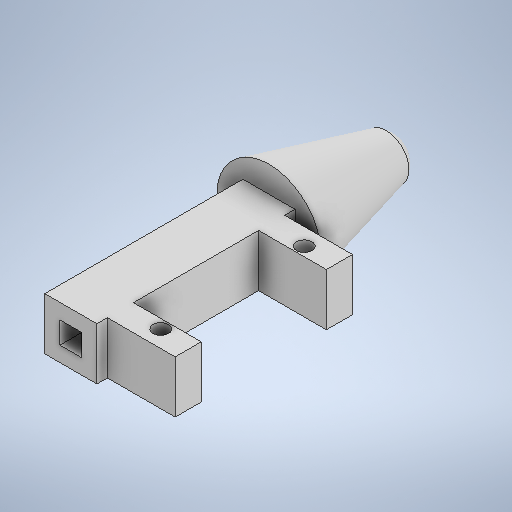
# Autodesk Inventor part: fot
Saved by Autodesk Inventor 2025.1 (Build 291241020, 241B)
## iProperties
Created: 2024-10-04
Part Number: fot
Material: Generic
Document SubType Name: Modeling
Designer: morte
Density: 1 g/cm^3
Appearance: Default
Author: morte
Autodesk Inventor part; units mm, degrees
ref_plane "YZ Plane" through (0, 0, 0) normal (1, 0, 0) x (0, 1, 0)
ref_plane "XZ Plane" through (0, 0, 0) normal (0, 1, 0) x (-1, 0, 0)
sketch "Sketch1" plane through (0, 0, 0) normal (0, 0, 1) x (1, 0, 0)
  line L0 (3.15, -3.15) -> (-3.15, -3.15)
  line L1 (-3.15, -3.15) -> (-3.15, 3.15)
  line L2 (-3.15, 3.15) -> (3.15, 3.15)
  line L3 (3.15, 3.15) -> (3.15, -3.15)
  line L4 (3.15, -3.15) -> (-3.15, 3.15) construction
  line L5 (-3.15, -3.15) -> (3.15, 3.15) construction
  line L6 (5, -5) -> (-5, -5)
  line L7 (-5, -5) -> (-5, 5)
  line L8 (-5, 5) -> (5, 5)
  line L9 (5, 5) -> (5, -5)
  line L10 (5, -5) -> (-5, 5) construction
  line L11 (-5, -5) -> (5, 5) construction
  point P0 (0, 0)
  dimension "d0" = 6.3
  dimension "d1" = 6.3
  dimension "d2" = 10
  dimension "d3" = 10
  constraints: 24 end point, 4 midpoint, 4 parallel, 2 horizontal, 2 perpendicular
  measures "d0" distance of L1.end L2.end
  measures "d1" distance of L0.end L1.end
  measures "d2" distance of L7.end L8.end
  measures "d3" distance of L6.end L7.end
extrude "Extrusion1" add sketch "Sketch1" along normal mid plane 60
sketch "Sketch3" plane through (0, 0, 0) normal (1, 0, 0) x (0, 1, 0)
  line L0 (5, -30) -> (-5, -30) projected
  line L1 (0, -30) -> (0, -50)
  line L2 (0, -30) -> (10, -30)
  arc A0 (0, -55) -> (4.3301, -52.5) centre (0, -50) ccw
  line L3 (0, -55) -> (0, -30)
  line L4 (4.3301, -52.5) -> (10, -30)
  point P0 (0, 0)
  dimension "d19" = 20
  dimension "d20" = 10
  dimension "d21" = 10
  dimension "d22" = 5
  constraints: 8 end point, 2 point on circle, 1 centre point, 1 coincident, 1 midpoint, 1 perpendicular, 1 point on line, 1 vertical
  measures "d19" distance of L1.start L1.end
  measures "d20" distance of L1.start L2.end
  measures "d21" diameter of A0
  measures "d22" distance of L3.start L4.start
revolve "Revolution1" add sketch "Sketch3" angle 360 about axis through (0, 0, -30) along (0, 0, -1)
sketch "Sketch4" plane through (0, 0, 0) normal (0, 1, 0) x (-1, 0, 0)
  point P0 (0, 0)
sketch "Sketch5" plane through (0, 0, 0) normal (0, 1, 0) x (-1, 0, 0)
  line L0 (-5, -30) -> (-5, 30) projected
  line L1 (-5, 0) -> (-5, -23)
  line L2 (-5, 30) -> (-5, -30) projected
  line L3 (-5, 0) -> (-5, 1)
  line L4 (-5, 1) -> (-5, 6)
  line L5 (-5, 6) -> (-18, 6)
  line L6 (-5, -23) -> (-5, -28)
  line L7 (-5, -28) -> (-18, -28)
  line L8 (-18, -28) -> (-18, -23)
  line L9 (-18, -23) -> (-5, -23)
  line L10 (-5, 1) -> (-18, 1)
  line L11 (-18, 1) -> (-18, 6)
  point P0 (-5, 6)
  point P1 (-5, -28)
  point P2 (-5, -23)
  point P3 (-5, 1)
  dimension "d135" = 23
  dimension "d136" = 1
  dimension "d138" = 13
  dimension "d139" = 5
  dimension "d140" = 13
  dimension "d141" = 5
  dimension "d143" = 5
  constraints: 20 end point, 4 perpendicular, 4 point on line, 1 horizontal, 1 midpoint
  measures "d135" distance of L1.start L1.end
  measures "d136" distance of L1.start L3.end
  measures "d138" distance of L4.end L5.end
  measures "d139" distance of L1.end L6.end
  measures "d140" distance of L6.end L7.end
  measures "d141" distance of L7.end L8.end
  measures "d143" distance of L10.end L5.end
extrude "Extrusion2" add sketch "Sketch5" along normal mid plane 10
sketch "Sketch7" plane through (-5, -5, 30) normal (0, -1, 0) x (1, 0, 0)
  line L0 (10, 0) -> (10, -60) projected
  line L1 (23, -53) -> (10, -53) projected
  line L2 (10, -53) -> (10, -29) projected
  line L3 (10, -53) -> (10, -29)
  line L4 (10, -29) -> (10, -27.25)
  line L5 (10, -29) -> (23, -29) projected
  line L6 (10, -27.25) -> (10, -29)
  line L7 (10, -53) -> (10, -54.75)
  line L8 (10, -54.75) -> (17, -54.75)
  line L9 (10, -27.25) -> (17, -27.25)
  circle A0 centre (17, -54.75) radius 1.5
  circle A1 centre (17, -27.25) radius 1.5
  point P0 (10, -23.5)
  point P1 (10, -48.5)
  dimension "d144" = 24
  dimension "d145" = 1.75
  dimension "d146" = 1.75
  dimension "d147" = 7
  dimension "d148" = 7
  dimension "d149" = 3
  dimension "d150" = 3
  constraints: 12 end point, 2 centre point, 2 coincident, 2 collinear, 2 horizontal, 2 point on line
  measures "d144" distance of L1.end L2.end
  measures "d145" distance of L2.end L4.end
  measures "d146" distance of L1.end L7.end
  measures "d147" distance of L7.end L8.end
  measures "d148" distance of L4.end L9.end
  measures "d149" diameter of A0
  measures "d150" diameter of A1
extrude "Extrusion3" cut sketch "Sketch7" against normal through all
sketch "Sketch19" plane through (0, 0, 30) normal (0, 0, 1) x (1, 0, 0)
  line L0 (0, 0) -> (2.1, 0)
  line L1 (2.1, 0) -> (2.1, -2.1)
  line L2 (2.1, -2.1) -> (-2.1, -2.1)
  line L3 (-2.1, -2.1) -> (-2.1, 2.1)
  line L4 (-2.1, 2.1) -> (2.1, 2.1)
  line L5 (2.1, 2.1) -> (2.1, 0)
  line L6 (3.15, 3.15) -> (-3.15, 3.15) projected
  line L7 (2.1, 2.1) -> (3.15, 3.15)
  line L8 (3.15, -3.15) -> (3.15, 3.15) projected
  line L9 (3.15, 3.15) -> (3.15, -3.15)
  line L10 (3.15, -3.15) -> (-3.15, -3.15)
  line L11 (-3.15, -3.15) -> (-3.15, 3.15)
  line L12 (-3.15, 3.15) -> (3.15, 3.15)
  point P0 (-3.15, 3.15)
  dimension "d151" = 2.1
  dimension "d152" = 2.1
  dimension "d153" = 4.2
  dimension "d154" = 4.2
  constraints: 22 end point, 7 perpendicular, 2 point on line, 1 collinear, 1 horizontal, 1 parallel
  measures "d151" distance of L0.start L0.end
  measures "d152" distance of L0.end L1.end
  measures "d153" distance of L1.end L2.end
  measures "d154" distance of L2.end L3.end
extrude "Extrusion13" add sketch "Sketch19" against normal blind 80
ref_plane "Work Plane2" through (0, 0, -26) normal (0, 0, 1) x (1, 0, 0)
sketch "Sketch22" plane through (-5, -5, 30) normal (0, -1, 0) x (1, 0, 0)
  line L0 (0, -60) -> (0, 0) projected
  line L1 (10, -24) -> (23, -24) projected
  line L2 (-4.5508, 0) -> (19.955, 0)
  line L3 (19.955, 0) -> (19.955, -22)
  line L4 (19.955, -22) -> (-10.1203, -22)
  line L5 (-10.1203, -22) -> (-10.1203, 0)
  line L6 (-10.1203, 0) -> (19.955, 0)
  point P0 (5, -30)
  point P1 (0, -31)
  dimension "d176" = 22
  constraints: 10 end point, 3 perpendicular, 1 collinear, 1 horizontal, 1 point on line
  measures "d176" distance of L2.end L3.end
extrude "Extrusion16" cut sketch "Sketch22" against normal through all
body "Solid1"
